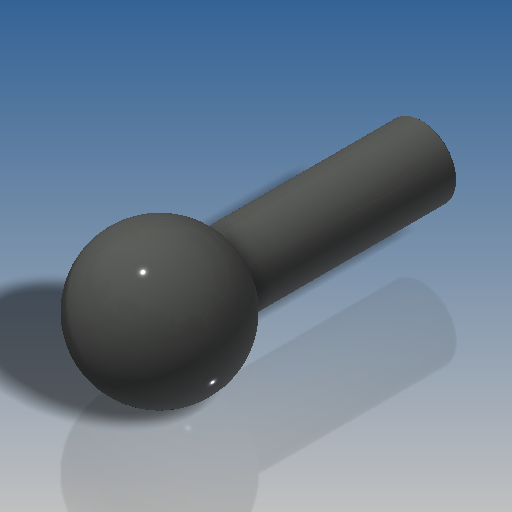
# Autodesk Inventor part: 22484-DkBluishGray
Saved by Autodesk Inventor 2018.3 (Build 223284000, 284)
## iProperties
Created: 2016-10-03
Part Number: 22484-DkBluishGray
Material: ABS Plastic
Document SubType Name: Modeling
Designer: D. Kohfeld
Density: 1.06 g/cm^3
Appearance: DkBluishGray
Mass: 0.222275 g
Surface Area: 2.20443 cm^2
Volume: 0.209694 cm^3
Author: D. Kohfeld
Autodesk Inventor part; units mm, degrees
ref_plane "YZ Plane" through (0, 0, 0) normal (1, 0, 0) x (0, 1, 0)
ref_plane "XZ Plane" through (0, 0, 0) normal (0, 1, 0) x (-1, 0, 0)
ref_plane "XY Plane" through (0, 0, 0) normal (0, 0, 1) x (1, 0, 0)
sketch "Sketch2" plane through (0, 0, 0) normal (1, 0, 0) x (0, 1, 0)
  line L0 (0, 3.2) -> (0, -12)
  line L1 (0, -12) -> (-1.6, -12)
  line L2 (-1.6, -12) -> (-1.6, -2.7713)
  arc A0 (0, 3.2) -> (-1.6, -2.7713) centre (0, 0) ccw
  dimension "d0" = 12
  dimension "d1" = 3.2
  dimension "d2" = 6.4
  constraints: 6 end point, 2 point on circle, 2 vertical, 1 centre point, 1 coincident, 1 horizontal, 1 point on line
  measures "d0" distance from line of L1 point (0, 0)
  measures "d1" diameter of L2 L0
  measures "d2" diameter of A0
revolve "Revolution1" add sketch "Sketch2" angle 360 about axis through (0, 0, 3.2) along (0, 0, -1)
fillet "Fillet1" radius 0.1 1 edges at (0, 1.6, -12)
equation "\"d1\" = rd"
equation "\"d4\" = lf"
equation "\"rd\" = 3.2"
equation "\"lf\" = 0.1"
body "Solid1"
